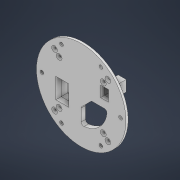
# Autodesk Inventor part: Cap
Saved by Autodesk Inventor 2022 (Build 260153000, 153)
## iProperties
Created: 2022-04-15
Part Number: Cap
Material: Generic
Document SubType Name: Modeling
Designer: dvorakj
Density: 1 g/cm^3
Appearance: Default
Author: dvorakj
Autodesk Inventor part; units mm, degrees
ref_plane "Work Plane1" through (0.0267, -0.004, 0) normal (0, 0, 1) x (1, 0, 0)
sketch "Sketch1" plane through (0.0267, -0.004, 0) normal (0, 0, 1) x (1, 0, 0)
  circle A0 centre (-57.7422, 0) radius 61.7422 projected
  point P0 (-0.0267, 0.004)
  point P1 (-57.7422, 0)
  constraints: 1 coincident
ref_plane "Work Plane2" through (-57.7155, -0.004, 0) normal (0, 1, 0) x (-1, 0, 0)
sketch "Sketch2" plane through (-57.7155, -0.004, 0) normal (0, 1, 0) x (-1, 0, 0)
  line L0 (0, 407.6086) -> (0, -419.6086) projected
  line L1 (61.7422, -55) -> (61.7422, 0)
  line L2 (46.7422, 0) -> (52.4903, 0) projected
  line L3 (52.2422, 0) -> (56.2422, 0) projected
  line L4 (56.3063, 0) -> (52.4903, 0) projected
  line L5 (57.7422, -35.7672) -> (57.7422, -56.2054)
  line L6 (57.7422, -35.7672) -> (57.7422, 0)
  line L7 (61.7422, 0) -> (61.7422, 3)
  line L8 (61.7422, 3) -> (0, 3)
  line L9 (57.7422, -3) -> (0, -3)
  line L10 (61.7422, 0) -> (57.7422, 0)
  dimension "d0" = 3
  dimension "d1" = 6
  constraints: 14 end point, 4 vertical, 3 point on line, 2 perpendicular, 1 horizontal, 4 other
  measures "d0" distance of L1.end L7.end
  measures "d1" distance between parallel lines of L8 L9
revolve "Revolution1" add sketch "Sketch2" angle 360 about axis through (-57.7155, -0.004, 407.6086) along (0, 0, -1)
sketch "Sketch4" plane through (-57.7155, -0.004, -3) normal (0, 0, -1) x (-1, 0, 0)
  circle A0 centre (-27.1211, -46.9752) radius 2 projected
  circle A1 centre (27.1211, -46.9752) radius 2 projected
  circle A2 centre (54.2422, 0) radius 2 projected
  circle A3 centre (27.1211, 46.9752) radius 2 projected
  circle A4 centre (-27.1211, 46.9752) radius 2 projected
  arc A5 (32.5606, -41.8117) -> (19.9296, -49.1042) centre (27.1211, -46.9752) ccw projected
  spline S0 degree 3 poles (39.6912, -41.9377) (39.2033, -42.3996) (38.6297, -42.7626) (37.3821, -43.2453) (36.72, -43.3629) (35.4002, -43.3347) (34.7552, -43.1937) (33.5548, -42.6678) (33.0125, -42.2877) (32.5606, -41.8117) knots 0 0 0 0 0.201555 0.201555 0.401366 0.401366 0.597736 0.597736 0.794788 0.794788 0.794788 0.794788 projected
  arc A6 (39.6912, -41.9377) -> (56.1648, -13.4047) centre (0, 0) ccw projected
  spline S1 degree 3 poles (52.4903, -7.2925) (53.1116, -7.4418) (53.6972, -7.7108) (54.7407, -8.4619) (55.1863, -8.9388) (55.8802, -10.0467) (56.1176, -10.67) (56.2902, -11.665) (56.3147, -12.0144) (56.2929, -12.7143) (56.2463, -13.0633) (56.1648, -13.4047) knots 0 0 0 0 0.191696 0.191696 0.385689 0.385689 0.58375 0.58375 0.68846 0.68846 0.793705 0.793705 0.793705 0.793705 projected
  arc A7 (52.4903, 7.2925) -> (52.4903, -7.2925) centre (54.2422, 0) ccw projected
  spline S2 degree 3 poles (56.1648, 13.4047) (56.3207, 12.7512) (56.3483, 12.073) (56.1426, 10.7512) (55.9134, 10.119) (55.2291, 8.9901) (54.7844, 8.5021) (53.7288, 7.7254) (53.1285, 7.4458) (52.4903, 7.2925) knots 0 0 0 0 0.201555 0.201555 0.401366 0.401366 0.597736 0.597736 0.794788 0.794788 0.794788 0.794788 projected
  arc A8 (56.1648, 13.4047) -> (39.6912, 41.9377) centre (0, 0) ccw projected
  spline S3 degree 3 poles (32.5606, 41.8117) (33.0006, 42.2751) (33.5263, 42.6478) (34.6986, 43.1759) (35.3343, 43.3233) (36.6408, 43.3703) (37.2993, 43.2642) (38.2473, 42.9162) (38.5621, 42.7628) (39.1574, 42.3939) (39.4363, 42.179) (39.6912, 41.9377) knots 0 0 0 0 0.191696 0.191696 0.385689 0.385689 0.58375 0.58375 0.68846 0.68846 0.793705 0.793705 0.793705 0.793705 projected
  arc A9 (19.9297, 49.1042) -> (32.5606, 41.8117) centre (27.1211, 46.9752) ccw projected
  spline S4 degree 3 poles (16.4735, 55.3425) (17.1175, 55.1508) (17.7186, 54.8356) (18.7605, 53.9965) (19.1934, 53.4819) (19.8289, 52.3248) (20.0292, 51.6957) (20.174, 50.3932) (20.116, 49.7335) (19.9297, 49.1042) knots 0 0 0 0 0.201555 0.201555 0.401366 0.401366 0.597736 0.597736 0.794788 0.794788 0.794788 0.794788 projected
  arc A10 (16.4735, 55.3425) -> (-16.4735, 55.3425) centre (0, 0) ccw projected
  spline S5 degree 3 poles (-19.9296, 49.1042) (-20.111, 49.7169) (-20.1709, 50.3585) (-20.0421, 51.6378) (-19.8519, 52.2621) (-19.2394, 53.417) (-18.8183, 53.9342) (-18.0429, 54.5812) (-17.7526, 54.7771) (-17.1355, 55.1082) (-16.81, 55.2423) (-16.4735, 55.3425) knots 0 0 0 0 0.191696 0.191696 0.385689 0.385689 0.58375 0.58375 0.68846 0.68846 0.793705 0.793705 0.793705 0.793705 projected
  arc A11 (-32.5606, 41.8117) -> (-19.9296, 49.1042) centre (-27.1211, 46.9752) ccw projected
  spline S6 degree 3 poles (-39.6912, 41.9377) (-39.2033, 42.3996) (-38.6297, 42.7626) (-37.3821, 43.2453) (-36.72, 43.3629) (-35.4002, 43.3347) (-34.7552, 43.1937) (-33.5548, 42.6678) (-33.0125, 42.2877) (-32.5606, 41.8117) knots 0 0 0 0 0.201555 0.201555 0.401366 0.401366 0.597736 0.597736 0.794788 0.794788 0.794788 0.794788 projected
  arc A12 (-39.6912, 41.9377) -> (-56.1648, 13.4047) centre (0, 0) ccw projected
  spline S7 degree 3 poles (-52.4903, 7.2925) (-53.1116, 7.4418) (-53.6972, 7.7108) (-54.7407, 8.4619) (-55.1863, 8.9388) (-55.8802, 10.0467) (-56.1176, 10.67) (-56.2902, 11.665) (-56.3147, 12.0144) (-56.2929, 12.7143) (-56.2463, 13.0633) (-56.1648, 13.4047) knots 0 0 0 0 0.191696 0.191696 0.385689 0.385689 0.58375 0.58375 0.68846 0.68846 0.793705 0.793705 0.793705 0.793705 projected
  arc A13 (-52.4903, -7.2925) -> (-52.4903, 7.2925) centre (-54.2422, 0) ccw projected
  spline S8 degree 3 poles (-56.1648, -13.4047) (-56.3207, -12.7512) (-56.3483, -12.073) (-56.1426, -10.7512) (-55.9134, -10.119) (-55.2291, -8.9901) (-54.7844, -8.5021) (-53.7288, -7.7254) (-53.1285, -7.4458) (-52.4903, -7.2925) knots 0 0 0 0 0.201555 0.201555 0.401366 0.401366 0.597736 0.597736 0.794788 0.794788 0.794788 0.794788 projected
  arc A14 (-56.1648, -13.4047) -> (-39.6912, -41.9377) centre (0, 0) ccw projected
  spline S9 degree 3 poles (-32.5606, -41.8117) (-33.0006, -42.2751) (-33.5263, -42.6478) (-34.6986, -43.1759) (-35.3343, -43.3233) (-36.6408, -43.3703) (-37.2993, -43.2642) (-38.2473, -42.9162) (-38.5621, -42.7628) (-39.1574, -42.3939) (-39.4363, -42.179) (-39.6912, -41.9377) knots 0 0 0 0 0.191696 0.191696 0.385689 0.385689 0.58375 0.58375 0.68846 0.68846 0.793705 0.793705 0.793705 0.793705 projected
  arc A15 (-19.9297, -49.1042) -> (-32.5606, -41.8117) centre (-27.1211, -46.9752) ccw projected
  spline S10 degree 3 poles (-16.4735, -55.3425) (-17.1175, -55.1508) (-17.7186, -54.8356) (-18.7605, -53.9965) (-19.1934, -53.4819) (-19.8289, -52.3248) (-20.0292, -51.6957) (-20.174, -50.3932) (-20.116, -49.7335) (-19.9297, -49.1042) knots 0 0 0 0 0.201555 0.201555 0.401366 0.401366 0.597736 0.597736 0.794788 0.794788 0.794788 0.794788 projected
  arc A16 (-16.4735, -55.3425) -> (16.4735, -55.3425) centre (0, 0) ccw projected
  spline S11 degree 3 poles (19.9296, -49.1042) (20.111, -49.7169) (20.1709, -50.3585) (20.0421, -51.6378) (19.8519, -52.2621) (19.2394, -53.417) (18.8183, -53.9342) (18.0429, -54.5812) (17.7526, -54.7771) (17.1355, -55.1082) (16.81, -55.2423) (16.4735, -55.3425) knots 0 0 0 0 0.191696 0.191696 0.385689 0.385689 0.58375 0.58375 0.68846 0.68846 0.793705 0.793705 0.793705 0.793705 projected
  circle A17 centre (-54.2422, 0) radius 2 projected
  circle A18 centre (0, 0) radius 61.7422 projected
  circle A19 centre (0, 0) radius 57.7422 projected
  point P0 (-57.7155, 0.004)
  point P1 (-39.6912, -41.9377)
  point P2 (-56.1648, 13.4047)
  point P3 (-16.4735, 55.3425)
  point P4 (39.6912, 41.9377)
  point P5 (56.1648, -13.4047)
  point P6 (16.4735, -55.3425)
ref_plane "Work Plane3" through (-119.4578, -61.7463, 0) normal (0, 0, 1) x (1, 0, 0)
extrude "Extrusion1" cut sketch "Sketch4" against normal up to surface (3 mm away) contours A0 | A1 | A2 | A3 | A4 | S0 A19 S11 A5 | S1 A7 S2 A19 | A19 S9 A15 S10 | A19 S7 A13 S8 | S3 A9 S4 A19 | A19 S5 A11 S6 | A17
sketch "Sketch5" plane through (-57.7155, -0.004, 3) normal (0, 0, 1) x (1, 0, 0)
  line L0 (-81.5245, 0) -> (93.5003, 0)
  circle A0 centre (0, 0) radius 61.7422 projected
  line L1 (-36.7696, -36.7696) -> (0, 0)
  circle A1 centre (-54.2422, 0) radius 2 projected
  circle A2 centre (0, 0) radius 54.2422
  circle A3 centre (-36.7696, -36.7696) radius 1.5
  circle A4 centre (-30.4056, -30.4056) radius 1.5
  point P0 (57.7155, 0.004)
  point P1 (36.7696, -36.7696)
  point P2 (36.7696, 36.7696)
  point P3 (-36.7696, 36.7696)
  point P4 (-0.4881, 0.3555)
  dimension "d7" = 360
  dimension "d9" = 45
  dimension "d10" = 3
  dimension "d11" = 3
  dimension "d12" = 9
  dimension "d13" = 52
  constraints: 4 end point, 3 coincident, 2 centre point, 2 point on line, 1 horizontal, 1 horizontal alignment, 8 other
  measures "d9" angle of L0 L1
  measures "d10" diameter of A3
  measures "d11" diameter of A4
  measures "d12" distance of A3.centre A4.centre
  measures "d13" distance of L1.start L1.end
extrude "Extrusion2" cut sketch "Sketch5" against normal blind 10 contours A3 | A4 L1 | L1 A4
fillet "Fillet1" radius 2.5 4 edges at (-95.985, -36.7736, -3) (-95.985, -36.7736, 3) (-89.6211, -30.4096, -3) (-89.6211, -30.4096, 3)
pattern_circular "Circular Pattern1" count 4 over 360 about axis through (-57.7155, -0.004, 1.5) along (0, 0, -1) of "Extrusion2", "Fillet1"
sketch "Sketch6" plane through (-57.7155, -0.004, 3) normal (0, 0, 1) x (1, 0, 0)
  line L0 (-18.9694, -21.0591) -> (-32.9694, -21.0591) projected
  line L1 (-32.9694, -21.0591) -> (-32.9694, 2.9409) projected
  line L2 (-18.9694, 2.9409) -> (-18.9694, -21.0591) projected
  line L3 (-32.9694, 2.9409) -> (-18.9694, 2.9409) projected
  point P0 (57.7155, 0.004)
extrude "Extrusion3" cut sketch "Sketch6" against normal blind 10
chamfer "Chamfer1" distance 2 angle 70 4 edges at (-76.6849, -9.0632, 3) (-83.6849, 2.9368, 3) (-90.6849, -9.0632, 3) (-83.6849, -21.0632, 3) measured on face at (-45.1453, 1.0596, 3)
sketch "Sketch7" plane through (-57.7155, -0.004, -3) normal (0, 0, -1) x (-1, 0, 0)
  line L0 (32.9694, 2.9409) -> (32.9694, -21.0591) projected
  line L1 (32.9694, -21.0591) -> (18.9694, -21.0591) projected
  line L2 (18.9694, -21.0591) -> (18.9694, 2.9409) projected
  line L3 (18.9694, 2.9409) -> (32.9694, 2.9409) projected
  line L4 (16.9694, -23.0591) -> (34.9694, -23.0591)
  line L5 (34.9694, -23.0591) -> (34.9694, 4.9409)
  line L6 (34.9694, 4.9409) -> (16.9694, 4.9409)
  line L7 (16.9694, 4.9409) -> (16.9694, -23.0591)
  point P0 (-57.7155, 0.004)
  dimension "d25" = 2
  constraints: 8 end point, 3 other
  measures "d25" distance between parallel lines of L1 L4
extrude "Extrusion4" add sketch "Sketch7" along normal blind 12
chamfer "Chamfer2" distance 1.5 angle 70 4 edges at (-76.6849, -9.0632, -15) (-90.6849, -9.0632, -15) (-83.6849, 2.9368, -15) (-83.6849, -21.0632, -15) measured on face at (-92.0182, -5.0632, -15)
sketch "Sketch11" plane through (-57.7155, -0.004, 3) normal (0, 0, 1) x (1, 0, 0)
  line L0 (28.268, 23.8945) -> (36.268, 23.8945)
  line L1 (36.268, 23.8945) -> (36.268, 11.8945)
  line L2 (36.268, 11.8945) -> (28.268, 11.8945)
  line L3 (28.268, 11.8945) -> (28.268, 23.8945)
  line L4 (26.768, 25.3945) -> (37.768, 25.3945)
  line L5 (37.768, 25.3945) -> (37.768, 10.3945)
  line L6 (37.768, 10.3945) -> (26.768, 10.3945)
  line L7 (26.768, 10.3945) -> (26.768, 25.3945)
  point P0 (57.7155, 0.004)
  dimension "d34" = 1.5
  dimension "d39" = 12
  dimension "d40" = 8
  constraints: 16 end point, 4 parallel, 2 perpendicular, 1 horizontal, 3 other
  measures "d34" distance between parallel lines of L3 L7
  measures "d39" distance of L0.end L1.end
  measures "d40" distance of L1.end L2.end
extrude "Extrusion5" add sketch "Sketch11" against normal blind 24.25
extrude "Extrusion6" cut sketch "Sketch11" against normal blind 9.5 contours L0 L1 L2 L3
chamfer "Chamfer3" distance 1.5 angle 70 4 edges at (-25.4475, 11.8904, 3) (-21.4475, 17.8904, 3) (-29.4475, 17.8904, 3) (-25.4475, 23.8904, 3) measured on face at (-44.6983, -3.5294, 3)
chamfer "Chamfer4" distance 1 angle 70 4 edges at (-25.4475, 11.8904, -21.25) (-21.4475, 17.8904, -21.25) (-29.4475, 17.8904, -21.25) (-25.4475, 23.8904, -21.25) measured on face at (-30.4475, 19.8904, -21.25)
sketch "Sketch12" plane through (-57.7155, -0.004, 3) normal (0, 0, 1) x (1, 0, 0)
  circle A0 centre (-54.2422, 0) radius 2 projected
  point P0 (57.7155, 0.004)
  constraints: 1 coincident
hole "Hole1" at (-111.9577, -0.004, 3) direction (0, 0, -1) diameter 3.4 end through all countersink diameter 5 countersink angle 90
pattern_circular "Circular Pattern2" count 6 over 360 about axis through (-57.7155, -0.004, 1.5) along (0, 0, -1) of "Hole1"
sketch "Sketch13" plane through (-57.7155, -0.004, 3) normal (0, 0, 1) x (1, 0, 0)
  circle A0 centre (0, 0) radius 35.7422
  line L0 (0, -35.7422) -> (0, -14.1421)
  line L1 (0, -14.1421) -> (14.1421, 0)
  line L2 (14.1421, 0) -> (35.7422, 0)
  circle A1 centre (0, 0) radius 61.7422 projected
  dimension "d57" = 135
  dimension "d58" = 10
  dimension "d59" = 26
  constraints: 6 end point, 2 point on circle, 1 centre point, 1 coincident, 1 horizontal, 1 horizontal alignment, 1 vertical, 1 vertical alignment
  measures "d57" angle of L0 L1
  measures "d58" distance from line of A0.centre L1
  measures "d59" radial gap between concentric circles of A1 A0
extrude "Extrusion7" cut sketch "Sketch13" against normal blind 9.5 contours A0 L0 L1 L2 picked at (12.1423, -14.0288)
fillet "Fillet2" radius 3.5 4 edges at (-57.7155, -35.7463, 0) (-57.7155, -14.1462, 0) (-43.5734, -0.004, 0) (-21.9733, -0.004, 0)
sketch "Sketch14" plane through (-57.7155, -0.004, -3) normal (0, 0, -1) x (-1, 0, 0)
  circle A0 centre (-36.7696, -36.7696) radius 4 projected
  circle A1 centre (-30.4056, -30.4056) radius 4 projected
  line L0 (-36.7696, -36.7696) -> (-30.4056, -30.4056)
  line L1 (-33.9411, -26.8701) -> (-26.8701, -33.9411)
  point P0 (-57.7155, 0.004)
  dimension "d64" = 10
  constraints: 4 end point, 1 midpoint, 1 perpendicular
  measures "d64" distance of L1.start L1.end
ref_plane "Work Plane7" through (-27.3099, -30.4096, -3) normal (-0.7071, -0.7071, 0) x (0.7071, -0.7071, 0)
sketch "Sketch15" plane through (-27.3099, -30.4096, -3) normal (-0.7071, -0.7071, 0) x (0.7071, -0.7071, 0)
  line L0 (10.5, 2.5) -> (7.5, 2.5) projected
  line L1 (5, 0) -> (13, 0) projected
  line L2 (1.5, 2.5) -> (-1.5, 2.5) projected
  line L3 (-4, 0) -> (4, 0) projected
  circle A0 centre (4.5, 0.4) radius 1.1
  point P0 (-2.1918, 3)
  dimension "d65" = 2.2
  dimension "d66" = 0.6403
  dimension "d67" = 0.6403
  dimension "d70" = 0.4
  constraints: 1 centre point
  measures "d65" diameter of A0
  measures "d66" distance of L1.start A0.centre
  measures "d67" distance of A0.centre L3.end
  measures "d70" distance from line of L3 A0.centre
extrude "Extrusion8" cut sketch "Sketch15" along normal mid plane 20.75
pattern_circular "Circular Pattern3" count 4 over 360 about axis through (-57.7155, -0.004, 1.5) along (0, 0, -1) of "Extrusion8"
equation "\"d66\" = d67"
body "Solid1"
